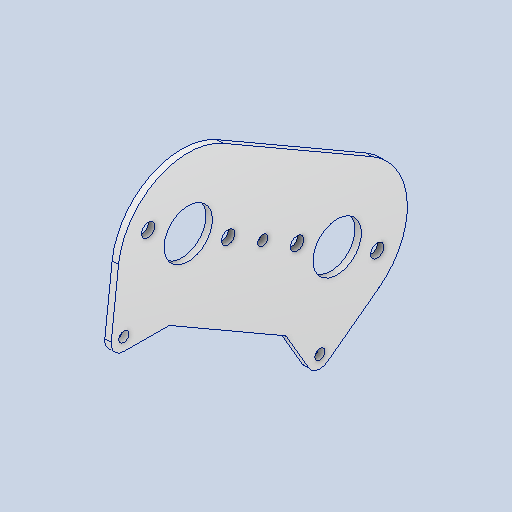
# Autodesk Inventor part: belt_liner_v5_Plate_15
Saved by Autodesk Inventor 2025.2 (Build 292293000, 293)
## iProperties
Created: 2025-03-06
Part Number: belt_liner_v5_Plate_15
Material: アルミニウム 6061
Document SubType Name: Modeling
Designer: haruy
Density: 2.7 g/cm^3
Appearance: アルミニウム - フラット
Author: haruy
Autodesk Inventor part; units mm, degrees
ref_plane "YZ Plane" through (0, 0, 0) normal (1, 0, 0) x (0, 1, 0)
ref_plane "XZ Plane" through (0, 0, 0) normal (0, 1, 0) x (-1, 0, 0)
ref_plane "XY Plane" through (0, 0, 0) normal (0, 0, 1) x (1, 0, 0)
derived "belt_liner_v5_Plate_14.ipt"
sketch "スケッチ1" plane through (300, 0, 0) normal (1, 0, 0) x (0, 1, 0)
  circle A0 centre (0, 0) radius 22.36 construction
  circle A1 centre (742.400277, -428.625) radius 23.875 construction
  line L0 (0, 0) -> (0, -985.832038)
  line L1 (0, 0) -> (742.400277, -428.625) construction
  line L2 (-48.743262, -24.425807) -> (-56.243262, -37.416188)
  line L3 (-56.243262, -37.416188) -> (725.777678, -488.916188)
  line L4 (725.777678, -488.916188) -> (733.277678, -475.925807)
  line L5 (733.277678, -475.925807) -> (-48.743262, -24.425807) construction
  line L6 (-44.122546, 123.258417) -> (-44.122546, 123.258417)
  line L7 (0, -985.832038) -> (0, 0)
  circle A2 centre (0, 0) radius 12.5
  circle A3 centre (0, 0) radius 15 construction
  line L8 (0, 0) -> (0, 0)
  circle A4 centre (0, 0) radius 24.06 construction
  line L9 (0, 0) -> (0, 0)
  line L10 (0, 0) -> (0, 0)
  line L11 (-48.743262, -24.425807) -> (-46.243262, -20.095679)
  circle A5 centre (742.400277, -428.625) radius 5 construction
  line L12 (733.277678, -475.925807) -> (707.296915, -460.925807)
  line L13 (707.296915, -460.925807) -> (709.796915, -456.595679)
  line L14 (709.796915, -456.595679) -> (735.777678, -471.595679)
  line L15 (735.777678, -471.595679) -> (733.277678, -475.925807)
  circle A6 centre (738.07015, -426.125) radius 5.1
  line L16 (742.400277, -428.625) -> (509.094258, -293.925707)
  circle A7 centre (759.720785, -438.625) radius 5.1
  line L17 (740.62015, -421.70827) -> (762.270785, -434.20827)
  line L18 (735.52015, -430.54173) -> (757.170785, -443.04173)
  circle A8 centre (742.400277, -428.625) radius 22.175 construction
  circle A9 centre (738.07015, -426.125) radius 10.1 construction
  circle A10 centre (759.720785, -438.625) radius 10.1 construction
  line L19 (743.12015, -417.378143) -> (764.770785, -429.878143) construction
  line L20 (733.02015, -434.871857) -> (754.670785, -447.371857) construction
  line L21 (743.12015, -417.378143) -> (730.659838, -410.184179) construction
  line L22 (729.323294, -421.075) -> (734.373294, -412.328143) construction
  line L23 (764.770785, -429.878143) -> (770.933518, -433.436199) construction
  line L24 (770.933518, -433.436199) -> (771.269456, -433.630153)
  line L25 (754.670785, -447.371857) -> (764.770785, -429.878143)
  line L26 (764.770785, -429.878143) -> (773.43104, -434.878143)
  line L27 (773.43104, -434.878143) -> (763.33104, -452.371857)
  line L28 (763.33104, -452.371857) -> (754.670785, -447.371857) construction
  circle A11 centre (725.867423, -468.760743) radius 1.5
  circle A12 centre (0, 0) radius 30 construction
  circle A13 centre (742.400277, -428.625) radius 6 construction
  circle A14 centre (0, 0) radius 24.06 construction
  circle A15 centre (0, 0) radius 24.06 construction
  circle A16 centre (742.400277, -428.625) radius 24.06
  line L29 (754.430277, -407.788429) -> (12.03, 20.836571) construction
  circle A17 centre (725.859192, -419.075) radius 4
  circle A18 centre (725.859192, -419.075) radius 1.5
  circle A19 centre (742.400277, -428.625) radius 18.525 construction
  circle A20 centre (748.98688, -417.41667) radius 4
  line L30 (737.43688, -437.421857) -> (742.48688, -428.675)
  circle A21 centre (748.98688, -417.41667) radius 1.5
  line L31 (734.373294, -412.328143) -> (737.823294, -406.352568) construction
  line L32 (737.823294, -406.352568) -> (776.88104, -428.902568)
  line L33 (773.43104, -434.878143) -> (776.88104, -428.902568)
  line L34 (737.823294, -406.352568) -> (723.650341, -415.740187)
  circle A22 centre (735.98688, -439.93333) radius 4
  circle A23 centre (735.98688, -439.93333) radius 1.5
  line L35 (720.823294, -435.797432) -> (759.88104, -458.347432)
  line L36 (763.33104, -452.371857) -> (759.88104, -458.347432)
  line L37 (720.823294, -435.797432) -> (721.866734, -418.829485)
  circle A24 centre (717.207169, -463.760743) radius 1.5
  circle A25 centre (742.400277, -428.625) radius 34.06
  circle A26 centre (742.48688, -428.675) radius 8.5
  line L38 (-57.983643, -13.420997) -> (-72.983643, -13.420997)
  line L39 (-72.983643, -13.420997) -> (-72.983643, -278.420997)
  line L40 (-72.983643, -278.420997) -> (-57.983643, -278.420997)
  line L41 (-57.983643, -278.420997) -> (-57.983643, -13.420997)
  line L42 (327.016357, -263.420997) -> (-72.983643, -263.420997)
  line L43 (-72.983643, -263.420997) -> (-72.983643, -278.420997)
  line L44 (-72.983643, -278.420997) -> (327.016357, -278.420997)
  line L45 (327.016357, -278.420997) -> (327.016357, -263.420997)
  line L46 (297.016357, -263.420997) -> (297.016357, -278.420997)
  line L47 (327.016357, -278.420997) -> (361.189313, -278.420997)
  line L48 (361.189313, -278.420997) -> (368.689313, -265.430616)
  line L49 (-207.983643, 176.579003) -> (-227.983643, 176.579003)
  line L50 (-227.983643, 176.579003) -> (-227.983643, -413.420997)
  line L51 (-227.983643, -413.420997) -> (-207.983643, -413.420997)
  line L52 (-207.983643, -413.420997) -> (-207.983643, 176.579003)
  line L53 (-51.406932, -263.569248) -> (-53.919015, -273.248579)
  line L54 (-53.919015, -273.248579) -> (703.30995, -469.772746)
  line L55 (703.30995, -469.772746) -> (705.822033, -460.093415)
  line L56 (705.822033, -460.093415) -> (-51.406932, -263.569248)
  circle A27 centre (0, 0) radius 24.06 construction
  line L57 (1412.720372, 281.579003) -> (-606.636412, 281.579003)
  line L58 (1185.577585, -518.420997) -> (-909.401992, -518.420997)
  line L59 (9.772119, 46.925807) -> (885.323802, -458.574193) construction
  line L60 (885.323802, -458.574193) -> (892.823802, -445.583812)
  line L61 (892.823802, -445.583812) -> (17.272119, 59.916188)
  line L62 (17.272119, 59.916188) -> (9.772119, 46.925807)
  line L63 (32.427564, 51.166188) -> (872.472205, -433.833812)
  line L64 (872.472205, -433.833812) -> (876.222205, -427.338622)
  line L65 (876.222205, -427.338622) -> (36.177564, 57.661378)
  line L66 (36.177564, 57.661378) -> (32.427564, 51.166188)
  line L67 (36.177564, 57.661378) -> (94.894086, 23.761378)
  line L68 (94.894086, 23.761378) -> (97.644086, 28.524518)
  line L69 (97.644086, 28.524518) -> (38.927564, 62.424518)
  line L70 (38.927564, 62.424518) -> (36.177564, 57.661378)
  circle A28 centre (218.051935, 108.540734) radius 120
  line L71 (77.016357, 123.579003) -> (57.016357, 123.579003)
  line L72 (57.016357, 123.579003) -> (57.016357, 103.579003)
  line L73 (57.016357, 103.579003) -> (77.016357, 103.579003)
  line L74 (77.016357, 103.579003) -> (77.016357, 123.579003)
  line L75 (218.051935, 108.540734) -> (186.993649, 224.451833)
  line L76 (218.051935, 108.540734) -> (102.140835, 77.482448)
  line L77 (218.051935, 108.540734) -> (158.051935, 4.617685)
  line L78 (189.993649, 229.647985) -> (99.140835, 72.286296)
  line L79 (99.140835, 72.286296) -> (93.944683, 75.286296)
  line L80 (93.944683, 75.286296) -> (184.797497, 232.647985)
  line L81 (184.797497, 232.647985) -> (189.993649, 229.647985)
  line L82 (184.797497, 232.647985) -> (181.797497, 227.451833)
  line L83 (181.797497, 227.451833) -> (177.46737, 229.951833)
  line L84 (177.46737, 229.951833) -> (180.46737, 235.147985)
  line L85 (180.46737, 235.147985) -> (184.797497, 232.647985)
  line L86 (93.944683, 75.286296) -> (96.944683, 80.482448)
  line L87 (96.944683, 80.482448) -> (92.614556, 82.982448)
  line L88 (92.614556, 82.982448) -> (89.614556, 77.786296)
  line L89 (89.614556, 77.786296) -> (93.944683, 75.286296)
  line L90 (77.016357, 123.579003) -> (117.016357, 123.579003)
  line L91 (117.016357, 123.579003) -> (117.016357, 103.579003)
  line L92 (117.016357, 103.579003) -> (77.016357, 103.579003)
  line L93 (77.016357, 103.579003) -> (77.016357, 123.579003)
  circle A29 centre (218.051935, 108.540734) radius 132.068148
  line L94 (103.677564, 174.574808) -> (38.927564, 62.424518)
  line L95 (32.427564, 51.166188) -> (11.695064, 15.256444) construction
  line L96 (11.695064, 15.256444) -> (20.355318, 10.256444) construction
  line L97 (20.355318, 10.256444) -> (41.087818, 46.166188) construction
  line L98 (41.087818, 46.166188) -> (32.427564, 51.166188)
  line L99 (152.017861, -5.833637) -> (158.051935, 4.617685)
  line L100 (152.017861, -5.833637) -> (20.355318, 10.256444) construction
  line L101 (74.812117, 3.601443) -> (78.312117, 9.663621)
  line L102 (78.312117, 9.663621) -> (92.571148, 1.431166)
  line L103 (181.797497, 227.451833) -> (154.291131, 210.199771)
  line L104 (96.944683, 80.482448) -> (98.132224, 112.92969)
  line L105 (99.140835, 72.286296) -> (116.392897, 44.77993)
  line L106 (-324.983643, 281.579003) -> (-324.983643, -518.420997)
  line L107 (1175.016357, 281.579003) -> (1175.016357, -518.420997)
  line L108 (17.272119, 59.916188) -> (9.772119, 46.925807)
  line L109 (9.772119, 46.925807) -> (-3.218262, 54.425807)
  line L110 (-3.218262, 54.425807) -> (4.281738, 67.416188)
  line L111 (4.281738, 67.416188) -> (17.272119, 59.916188)
  line L112 (-3.218262, 54.425807) -> (-5.718262, 50.095679)
  line L113 (-5.718262, 50.095679) -> (22.427564, 33.845679)
  line L114 (22.427564, 33.845679) -> (24.927564, 38.175807)
  line L115 (24.927564, 38.175807) -> (-3.218262, 54.425807)
  line L116 (-48.743262, -24.425807) -> (-46.243262, -20.095679)
  line L117 (-46.243262, -20.095679) -> (5.718262, -50.095679) construction
  line L118 (5.718262, -50.095679) -> (3.218262, -54.425807) construction
  line L119 (3.218262, -54.425807) -> (-48.743262, -24.425807) construction
  line L120 (789.608636, -403.313017) -> (798.26889, -408.313017)
  line L121 (798.26889, -408.313017) -> (785.03639, -431.232379)
  line L122 (785.03639, -431.232379) -> (776.376136, -426.232379)
  line L123 (776.376136, -426.232379) -> (789.608636, -403.313017)
  line L124 (885.323802, -458.574193) -> (882.823802, -462.904321)
  line L125 (882.823802, -462.904321) -> (856.84304, -447.904321)
  line L126 (856.84304, -447.904321) -> (859.34304, -443.574193)
  line L127 (859.34304, -443.574193) -> (885.323802, -458.574193)
  line L128 (7.607055, 48.175807) -> (11.937182, 45.675807)
  line L129 (11.937182, 45.675807) -> (19.437182, 58.666188)
  line L130 (19.437182, 58.666188) -> (15.107055, 61.166188)
  line L131 (15.107055, 61.166188) -> (7.607055, 48.175807)
  line L132 (19.437182, 58.666188) -> (14.437182, 50.005934)
  line L133 (14.437182, 50.005934) -> (24.829487, 44.005934)
  line L134 (24.829487, 44.005934) -> (29.829487, 52.666188)
  line L135 (29.829487, 52.666188) -> (19.437182, 58.666188)
  line L136 (931.223149, -485.074193) -> (935.553276, -487.574193)
  line L137 (935.553276, -487.574193) -> (951.553276, -459.861381)
  line L138 (951.553276, -459.861381) -> (947.223149, -457.361381)
  line L139 (947.223149, -457.361381) -> (931.223149, -485.074193)
  line L140 (944.473149, -462.12452) -> (934.973149, -478.579003)
  line L141 (934.973149, -478.579003) -> (919.384691, -469.579003)
  line L142 (919.384691, -469.579003) -> (928.884691, -453.12452)
  line L143 (928.884691, -453.12452) -> (944.473149, -462.12452)
  line L144 (924.134691, -461.351762) -> (939.723149, -470.351762)
  line L145 (926.634691, -457.021635) -> (921.634691, -465.681889)
  line L146 (921.634691, -465.681889) -> (882.663548, -443.181889)
  line L147 (882.663548, -443.181889) -> (887.663548, -434.521635)
  line L148 (887.663548, -434.521635) -> (926.634691, -457.021635)
  line L149 (888.913548, -432.356571) -> (881.413548, -445.346952)
  line L150 (881.413548, -445.346952) -> (874.485345, -441.346952)
  line L151 (874.485345, -441.346952) -> (881.985345, -428.356571)
  line L152 (881.985345, -428.356571) -> (888.913548, -432.356571)
  line L153 (31.079487, 54.831251) -> (23.579487, 41.84087)
  line L154 (23.579487, 41.84087) -> (30.507691, 37.84087)
  line L155 (30.507691, 37.84087) -> (38.007691, 50.831251)
  line L156 (38.007691, 50.831251) -> (31.079487, 54.831251)
  line L157 (16.937182, 54.336061) -> (27.329487, 48.336061)
  circle A30 centre (4.191992, 47.260743) radius 1.25
  circle A31 centre (12.852246, 42.260743) radius 1.25
  line L158 (17.272119, 59.916188) -> (9.772119, 46.925807)
  line L159 (885.323802, -458.574193) -> (882.823802, -462.904321)
  line L160 (882.823802, -462.904321) -> (933.053276, -491.904321)
  line L161 (933.053276, -491.904321) -> (935.553276, -487.574193)
  line L162 (935.553276, -487.574193) -> (885.323802, -458.574193)
  line L163 (375.016357, 281.579003) -> (375.016357, -518.420997)
  line L164 (38.927564, 62.424518) -> (41.427564, 66.754645)
  line L165 (41.427564, 66.754645) -> (100.144086, 32.854645)
  line L166 (100.144086, 32.854645) -> (97.644086, 28.524518)
  line L167 (97.644086, 28.524518) -> (38.927564, 62.424518)
  line L168 (97.724213, 18.663302) -> (115.044721, 8.663302)
  line L169 (115.044721, 8.663302) -> (117.544721, 12.993429)
  line L170 (117.544721, 12.993429) -> (100.224213, 22.993429)
  line L171 (100.224213, 22.993429) -> (97.724213, 18.663302)
  line L172 (116.294721, 10.828365) -> (98.974213, 20.828365)
  line L173 (327.016357, -263.420997) -> (335.208551, -263.420997)
  line L174 (335.208551, -263.420997) -> (342.708551, -250.430616)
  line L175 (-48.743262, -24.425807) -> (-56.243262, -37.416188)
  line L176 (-56.243262, -37.416188) -> (-77.893897, -24.916188)
  line L177 (-77.893897, -24.916188) -> (-70.393897, -11.925807)
  line L178 (-70.393897, -11.925807) -> (-48.743262, -24.425807)
  line L179 (-207.983643, -73.420997) -> (-72.983643, -73.420997) construction
  line L180 (-72.983643, -73.420997) -> (-72.983643, -93.420997)
  line L181 (-72.983643, -93.420997) -> (-207.983643, -93.420997) construction
  line L182 (-207.983643, -93.420997) -> (-207.983643, -73.420997)
  line L183 (-72.983643, -198.420997) -> (-207.983643, -198.420997) construction
  line L184 (-207.983643, -198.420997) -> (-207.983643, -218.420997)
  line L185 (-207.983643, -218.420997) -> (-72.983643, -218.420997) construction
  line L186 (-72.983643, -218.420997) -> (-72.983643, -198.420997)
  line L187 (-227.983643, -118.420997) -> (-207.983643, -118.420997)
  circle A32 centre (-30.172754, -32.260743) radius 1.25 construction
  circle A33 centre (-12.852246, -42.260743) radius 1.25 construction
  line L188 (-5.718262, 50.095679) -> (-46.243262, -20.095679)
  circle A34 centre (44.676915, 5.382686) radius 15 construction
  circle A35 centre (17.676915, -41.382686) radius 15 construction
  circle A36 centre (44.676915, 5.382686) radius 22
  circle A37 centre (17.676915, -41.382686) radius 22
  circle A38 centre (31.176915, -18) radius 3 construction
  line L189 (44.676915, 5.382686) -> (17.676915, -41.382686) construction
  circle A39 centre (26.744828, 25.567835) radius 3 construction
  circle A40 centre (-8.769981, -35.945618) radius 3 construction
  circle A41 centre (866.753294, -450.739257) radius 1.25
  circle A42 centre (875.413548, -455.739257) radius 1.25
  circle A43 centre (994.876722, -339.959266) radius 120
  line L190 (278.051935, 212.463782) -> (1054.876722, -236.036218)
  line L191 (-207.983643, -118.420997) -> (1175.016357, -118.420997)
  line L192 (-227.983643, -283.420997) -> (-207.983643, -283.420997)
  line L193 (-72.983643, -68.420997) -> (-92.983643, -68.420997)
  line L194 (-92.983643, -68.420997) -> (-92.983643, -88.420997)
  line L195 (-92.983643, -88.420997) -> (-72.983643, -88.420997)
  line L196 (-72.983643, -88.420997) -> (-72.983643, -68.420997)
  line L197 (-72.983643, -218.420997) -> (-92.983643, -218.420997)
  line L198 (-92.983643, -218.420997) -> (-92.983643, -238.420997)
  line L199 (-92.983643, -238.420997) -> (-72.983643, -238.420997)
  line L200 (-72.983643, -238.420997) -> (-72.983643, -218.420997)
  circle A44 centre (-28.727151, -34.637419) radius 15
  circle A45 centre (26.744828, 25.567835) radius 1.6
  circle A46 centre (31.176915, -18) radius 1.6
  circle A47 centre (-8.769981, -35.945618) radius 1.6
  circle A48 centre (44.676915, 5.382686) radius 7.6
  circle A49 centre (44.676915, 5.382686) radius 14.5
  circle A50 centre (37.426915, -7.174682) radius 2.1
  circle A51 centre (51.926915, 17.940054) radius 2.1
  circle A52 centre (17.676915, -41.382686) radius 7.6
  circle A53 centre (17.676915, -41.382686) radius 14.5
  circle A54 centre (24.926915, -28.825318) radius 2.1
  circle A55 centre (10.426915, -53.940054) radius 2.1
  circle A56 centre (-28.727151, -34.637419) radius 6.1
  circle A57 centre (-28.727151, -34.637419) radius 9
  circle A58 centre (-21.580715, -40.10811) radius 1.6
  circle A59 centre (-35.873586, -29.166728) radius 1.6
  circle A60 centre (26.744828, 25.567835) radius 4
  circle A61 centre (31.176915, -18) radius 4
  circle A62 centre (-8.769981, -35.945618) radius 4
  line L201 (27.340302, 29.523263) -> (27.340302, 29.523263)
  line L202 (27.202664, 29.541547) -> (47.195016, 27.238101)
  line L203 (63.729473, -5.617314) -> (36.729473, -52.382686)
  line L204 (22.74485, 25.581313) -> (22.677039, 5.456816)
  line L205 (25.624356, 16.382686) -> (-1.375644, -30.382686)
  line L206 (17.556098, -19.383018) -> (-28.809525, -19.637645) construction
  line L207 (-33.0766, -48.992986) -> (11.297722, -62.437517) construction
  line L208 (-10.781642, -32.488275) -> (6.612779, -22.3673)
  line L209 (-11.982398, -38.328972) -> (0.008621, -54.491133)
  line L210 (-92.983643, 143.579003) -> (-112.983643, 143.579003)
  line L211 (-112.983643, 143.579003) -> (-112.983643, -340.420997)
  line L212 (-112.983643, -340.420997) -> (-92.983643, -340.420997)
  line L213 (-92.983643, -340.420997) -> (-92.983643, 143.579003)
  line L214 (-98.670644, -321.246586) -> (-92.983643, -340.420997)
  line L215 (-92.983643, -340.420997) -> (762.327689, -86.741448)
  line L216 (762.327689, -86.741448) -> (756.640689, -67.567037)
  line L217 (756.640689, -67.567037) -> (-98.670644, -321.246586)
  line L218 (297.016357, -278.420997) -> (282.016357, -278.420997)
  line L219 (282.016357, -278.420997) -> (282.016357, -293.420997)
  line L220 (282.016357, -293.420997) -> (297.016357, -293.420997)
  line L221 (297.016357, -293.420997) -> (297.016357, -278.420997)
  line L222 (282.016357, -293.420997) -> (267.016357, -293.420997)
  line L223 (267.016357, -293.420997) -> (267.016357, -210.992417)
  line L224 (267.016357, -210.992417) -> (282.016357, -210.992417)
  line L225 (282.016357, -210.992417) -> (282.016357, -293.420997)
  line L226 (947.223149, -457.361381) -> (854.33083, -403.729976)
  circle A63 centre (257.889103, 85.540734) radius 120
  line L227 (-189.983643, 176.579003) -> (-189.983643, -384.012647)
  line L228 (-345.411643, 103.579003) -> (-345.411643, -457.361381)
  line L229 (-57.983643, -98.420997) -> (-92.983643, -98.420997)
  line L230 (218.051935, 108.540734) -> (218.051935, -11.459266)
  line L231 (218.051935, 108.540734) -> (218.051935, 228.540734)
  point P0 (730.659838, -410.184179)
  point P1 (-65.483643, -23.420997)
  point P2 (-65.483643, -270.920997)
  point P3 (317.016357, -270.920997)
  point P4 (307.016357, -270.920997)
  point P5 (347.610474, -261.920997)
  point P6 (356.270728, -266.920997)
  point P7 (-42.983643, -270.920997)
  point P8 (694.886661, -462.420997)
  point P9 (57.016357, 113.579003)
  point P10 (782.992386, -414.772698)
  point P11 (931.92892, -465.851762)
  point P12 (22.696769, 11.311957)
  point P13 (1.551943, -25.311957)
  point P14 (0, -54.479506)
  point P15 (274.516357, -220.992417)
extrude "押し出し1" add sketch "スケッチ1" against normal blind 2 contours L208 L205 L0 | L0 L205 A37 L209 A62 L208 | L205 L208 A37 L0 | L0 A37 L205 | A62 | L205 L204 A36 L203 A37 L208 | A37 L0 | L0 A37 | L205 A36 L204 | L204 A60 L202 A36 L205 | A60 | A36 | A49 A50 A51 | A53 A55 A54 | A61
fillet "フィレット1" radius 2 2 edges at (299, 22.6968, 11.312) (299, 1.5519, -25.312)
